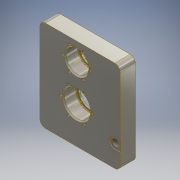
# Autodesk Inventor part: корпус_02
Saved by Autodesk Inventor 2016 (Build 200138000, 138)
## iProperties
Created: 2021-04-26
Part Number: корпус_02
Material: Типовые
Document SubType Name: Modeling
Designer: Лол
Density: 1 g/cm^3
Appearance: Титан — полированный
Author: Лол
Autodesk Inventor part; units mm, degrees
ref_plane "YZ Plane" through (0, 0, 0) normal (1, 0, 0) x (0, 1, 0)
ref_plane "XY Plane" through (0, 0, 0) normal (0, 0, 1) x (1, 0, 0)
ref_plane "РабПлоскость1" through (0, -12.5, 0) normal (0, 1, 0) x (-1, 0, 0)
sketch "Эскиз2" plane through (0, -12.5, 0) normal (0, 1, 0) x (-1, 0, 0)
  line L0 (100, 120) -> (-120, 120)
  line L1 (-120, 120) -> (-120, -130)
  line L2 (-120, -130) -> (100, -130)
  line L3 (100, -130) -> (100, 120)
  line L4 (144, 0) -> (-164, 0) projected
  line L5 (-164, 0) -> (144, 0) projected
  line L6 (0, -180) -> (0, 170) projected
  circle A0 centre (0, 70) radius 27
  circle A1 centre (0, -30) radius 31.5
  point P0 (0, 0)
  dimension "d10" = 120
  dimension "d11" = 130
  dimension "d12" = 120
  dimension "d13" = 100
  dimension "d14" = 70
  dimension "d15" = 30
  dimension "d16" = 63
  dimension "d17" = 54
  constraints: 8 end point, 2 centre point, 2 parallel, 2 point on line, 1 horizontal, 1 perpendicular
  measures "d10" distance between parallel lines of L4 L0
  measures "d11" distance between parallel lines of L2 L4
  measures "d12" distance between parallel lines of L6 L1
  measures "d13" distance between parallel lines of L3 L6
  measures "d14" distance from line of L4 A0.centre
  measures "d15" distance from line of A1.centre L4
  measures "d16" diameter of A1
  measures "d17" diameter of A0
extrude "Выдавливание2" add sketch "Эскиз2" against normal blind 42 contours L3 L4 A1 L6 A0 L0 | L6 A0 A1 L4 L1 L0 | L3 L2 L6 A1 L4 | L4 A1 L6 L2 L1
fillet "Сопряжение1" radius 15 4 edges at (120, -33.5, 120) (120, -33.5, -130) (-100, -33.5, 120) (-100, -33.5, -130)
sketch "Эскиз3" plane through (0, -12.5, 0) normal (0, 1, 0) x (1, 0, 0)
  line L0 (-85, -120) -> (105, -120) projected
  arc A0 (-100, -105) -> (-85, -120) centre (-85, -105) ccw construction
  line L1 (-100, 115) -> (-100, -105) projected
  arc A1 (-85, 130) -> (-100, 115) centre (-85, 115) ccw construction
  arc A2 (120, 115) -> (105, 130) centre (105, 115) ccw projected
  line L2 (120, -105) -> (120, 115) projected
  arc A3 (105, -120) -> (120, -105) centre (105, -105) ccw projected
  arc A4 (-85, 130) -> (-100, 115) centre (-85, 115) ccw projected
  line L3 (-100, 115) -> (-100, -105) projected
  arc A5 (-100, -105) -> (-85, -120) centre (-85, -105) ccw projected
  line L4 (-85, -120) -> (105, -120) projected
  arc A6 (105, -120) -> (120, -105) centre (105, -105) ccw projected
  line L5 (120, -105) -> (120, 115) projected
  arc A7 (120, 115) -> (105, 130) centre (105, 115) ccw projected
  line L6 (105, 130) -> (-85, 130) construction
  circle A8 centre (0, 30) radius 31.5 projected
  circle A9 centre (0, -70) radius 27 projected
  circle A10 centre (0, 30) radius 31.5 projected
  arc A11 (-94, -105) -> (-85, -114) centre (-85, -105) ccw
  arc A12 (105, -114) -> (114, -105) centre (105, -105) ccw
  line L7 (114, -105) -> (114, 115)
  arc A13 (114, 115) -> (105, 124) centre (105, 115) ccw
  line L8 (105, 124) -> (-85, 124)
  arc A14 (-85, 124) -> (-94, 115) centre (-85, 115) ccw
  line L9 (-94, 115) -> (-94, -105)
  arc A15 (27.534, -11.7358) -> (-27.534, -11.7358) centre (0, 30) ccw
  arc A16 (35.3716, -97.8182) -> (26.8965, -33.9226) centre (0, -70) ccw
  arc A17 (-26.8965, -33.9226) -> (-35.3716, -97.8182) centre (0, -70) ccw
  arc A18 (-26.8965, -33.9226) -> (-27.534, -11.7358) centre (-35.0001, -23.0529) ccw
  arc A19 (27.534, -11.7358) -> (26.8965, -33.9226) centre (35.0001, -23.0529) ccw
  line L10 (168.3492, 0) -> (-148.3492, 0) projected
  line L11 (0, 184.3492) -> (0, -174.3492) projected
  line L12 (-85, -114) -> (-43.2319, -114)
  line L13 (43.2319, -114) -> (105, -114)
  arc A20 (-43.2319, -114) -> (-35.3716, -97.8182) centre (-43.2319, -104) ccw
  arc A21 (35.3716, -97.8182) -> (43.2319, -114) centre (43.2319, -104) ccw
  point P0 (0, 0)
  dimension "d21" = 6
  dimension "d22" = 100
  dimension "d24" = 45
  dimension "d25" = 45
  dimension "d27" = 13.558
  dimension "d28" = 6
  dimension "d32" = 10
  dimension "d33" = 10
  dimension "d34" = 238
  dimension "d35" = 114
  dimension "d38" = 114
  constraints: 22 point on circle, 11 centre point, 10 end point, 9 tangent, 2 coincident, 1 equal radius, 3 other
  measures "d21" distance between parallel lines of L1 L9
  measures "d22" diameter of A15
  measures "d24" radius of A17
  measures "d25" radius of A16
  measures "d27" radius of A18
  measures "d28" distance between parallel lines of L0 L13
  measures "d32" radius of A20
  measures "d33" radius of A21
  measures "d34" distance between parallel lines of L12 L8
  measures "d35" distance between parallel lines of L11 L7
  measures "d38" distance between parallel lines of L10 L12
extrude "Выдавливание5" cut sketch "Эскиз3" against normal blind 34 contours L10 A15 A18 A17 A20 L12 A11 L9 | L9 A14 L8 L11 A15 L10 | L10 A15 L11 L8 A13 L7 | L7 A12 L13 A21 A16 A19 A15 L10
sketch "Эскиз4" plane through (0, -54.5, 0) normal (0, -1, 0) x (1, 0, 0)
  circle A0 centre (0, -30) radius 31.5 projected
  circle A1 centre (0, 70) radius 27 projected
  arc A2 (-100, -115) -> (-85, -130) centre (-85, -115) ccw projected
  line L0 (-85, -130) -> (105, -130) projected
  arc A3 (105, -130) -> (120, -115) centre (105, -115) ccw projected
  line L1 (120, -115) -> (120, 105) projected
  arc A4 (120, 105) -> (105, 120) centre (105, 105) ccw projected
  line L2 (105, 120) -> (-85, 120) projected
  arc A5 (-85, 120) -> (-100, 105) centre (-85, 105) ccw projected
  line L3 (-100, 105) -> (-100, -115) projected
  circle A6 centre (0, 70) radius 31
  circle A7 centre (0, -30) radius 36
  circle A8 centre (0, -30) radius 31.5
  circle A9 centre (0, 70) radius 27
  point P0 (0, 0)
  dimension "d41" = 62
  dimension "d42" = 72
  constraints: 4 centre point, 4 coincident, 2 concentric
  measures "d41" diameter of A6
  measures "d42" diameter of A7
extrude "Выдавливание7" cut sketch "Эскиз4" against normal blind 37 contours A6 | A7
sketch "Эскиз5" plane through (0, -12.5, 0) normal (0, 1, 0) x (1, 0, 0)
  arc A0 (105, -120) -> (120, -105) centre (105, -105) ccw projected
  arc A1 (-100, -105) -> (-85, -120) centre (-85, -105) ccw projected
  arc A2 (-85, 130) -> (-100, 115) centre (-85, 115) ccw projected
  arc A3 (120, 115) -> (105, 130) centre (105, 115) ccw projected
  arc A4 (-70, 115) -> (-94, 103) centre (-85, 115) ccw
  circle A5 centre (-85, -105) radius 15
  arc A6 (114, 103) -> (90, 115) centre (105, 115) ccw
  circle A7 centre (105, -105) radius 15
  line L0 (105, -114) -> (43.2319, -114) projected
  line L1 (114, 115) -> (114, -105) projected
  arc A8 (-94, -105) -> (-85, -114) centre (-85, -105) ccw projected
  line L2 (-43.2319, -114) -> (-85, -114) projected
  arc A9 (-43.2319, -114) -> (-35.3716, -97.8182) centre (-43.2319, -104) ccw projected
  arc A10 (-26.8965, -33.9226) -> (-35.3716, -97.8182) centre (0, -70) ccw projected
  arc A11 (-26.8965, -33.9226) -> (-27.534, -11.7358) centre (-35.0001, -23.0529) ccw projected
  arc A12 (27.534, -11.7358) -> (-27.534, -11.7358) centre (0, 30) ccw projected
  arc A13 (27.534, -11.7358) -> (26.8965, -33.9226) centre (35.0001, -23.0529) ccw projected
  arc A14 (35.3716, -97.8182) -> (26.8965, -33.9226) centre (0, -70) ccw projected
  arc A15 (35.3716, -97.8182) -> (43.2319, -114) centre (43.2319, -104) ccw projected
  line L3 (105, -114) -> (43.2319, -114) projected
  arc A16 (105, -114) -> (114, -105) centre (105, -105) ccw projected
  line L4 (114, 115) -> (114, -105) projected
  arc A17 (114, 115) -> (105, 124) centre (105, 115) ccw projected
  line L5 (-85, 124) -> (105, 124) projected
  arc A18 (-85, 124) -> (-94, 115) centre (-85, 115) ccw projected
  line L6 (-94, -105) -> (-94, 115) projected
  line L7 (-85, 124) -> (105, 124) projected
  line L8 (-94, -105) -> (-94, 115) projected
  line L9 (-43.2319, -114) -> (-85, -114) projected
  line L10 (-70, 115) -> (-70, 65)
  arc A19 (-94, 53) -> (-70, 65) centre (-85, 65) ccw
  line L11 (-100, 115) -> (-100, -105) projected
  line L12 (90, 115) -> (90, 65)
  arc A20 (90, 65) -> (114, 53) centre (105, 65) ccw
  line L13 (105, 65) -> (105, 115) construction
  line L14 (120, -105) -> (120, 115) projected
  point P0 (0, 0)
  dimension "d117" = 50
  dimension "d118" = 50
  constraints: 8 point on circle, 6 centre point, 6 end point, 6 equal radius, 4 coincident, 4 point on line, 3 vertical, 2 tangent, 1 parallel
  measures "d117" distance of L10.end L10.start
  measures "d118" distance of A2.centre A19.centre
extrude "Выдавливание8" add sketch "Эскиз5" against normal blind 37 contours A7 L0 A16 L1 A0 | A7 L1 A16 L0 | A6 L1 A17 L5 A3 | A20 L12 A6 L5 A17 L1 | L5 A18 L6 A4 A2 | A4 L10 A19 L6 A18 L5 | A5 L6 A8 L2 A1 | A5 L2 A8 L6
fillet "Сопряжение2" radius 15 2 edges at (-73, -29.5, 114) (93, -29.5, -124)
fillet "Сопряжение3" radius 5 6 edges at (114, -29.5, 93) (93, -29.5, 114) (-94, -29.5, 93) (-73, -29.5, -124) (-94, -29.5, -53) (114, -29.5, -53)
sketch "Эскиз6" plane through (0, -12.5, 0) normal (0, 1, 0) x (1, 0, 0)
  line L0 (85.4041, -114) -> (43.2319, -114) projected
  arc A0 (35.3716, -97.8182) -> (43.2319, -114) centre (43.2319, -104) ccw projected
  arc A1 (35.3716, -97.8182) -> (26.8965, -33.9226) centre (0, -70) ccw projected
  arc A2 (27.534, -11.7358) -> (26.8965, -33.9226) centre (35.0001, -23.0529) ccw projected
  arc A3 (27.534, -11.7358) -> (-27.534, -11.7358) centre (0, 30) ccw projected
  arc A4 (-26.8965, -33.9226) -> (-27.534, -11.7358) centre (-35.0001, -23.0529) ccw projected
  arc A5 (-26.8965, -33.9226) -> (-35.3716, -97.8182) centre (0, -70) ccw projected
  arc A6 (-43.2319, -114) -> (-35.3716, -97.8182) centre (-43.2319, -104) ccw projected
  line L1 (-43.2319, -114) -> (-55.6061, -114) projected
  arc A7 (-70.3031, -102) -> (-55.6061, -114) centre (-55.6061, -99) ccw projected
  arc A8 (-70.3031, -102) -> (-88, -90.3031) centre (-85, -105) ccw projected
  arc A9 (-94, -85.4041) -> (-88, -90.3031) centre (-89, -85.4041) ccw projected
  line L2 (-94, -85.4041) -> (-94, 45.4041) projected
  arc A10 (-70, 115) -> (-70.3031, 118) centre (-85, 115) ccw projected
  arc A11 (-65.4041, 124) -> (-70.3031, 118) centre (-65.4041, 119) ccw projected
  line L3 (-65.4041, 124) -> (75, 124) projected
  arc A12 (90, 109) -> (75, 124) centre (75, 109) ccw projected
  line L4 (114, 45.4041) -> (114, -85.4041) projected
  arc A13 (108, -90.3031) -> (114, -85.4041) centre (109, -85.4041) ccw projected
  arc A14 (108, -90.3031) -> (90.3031, -108) centre (105, -105) ccw projected
  arc A15 (85.4041, -114) -> (90.3031, -108) centre (85.4041, -109) ccw projected
  circle A16 centre (0, -70) radius 27 projected
  circle A17 centre (0, 30) radius 31.5 projected
  arc A18 (105, -120) -> (120, -105) centre (105, -105) ccw projected
  line L5 (120, -105) -> (120, 115) projected
  arc A19 (120, 115) -> (105, 130) centre (105, 115) ccw projected
  line L6 (105, 130) -> (-85, 130) projected
  arc A20 (-85, 130) -> (-100, 115) centre (-85, 115) ccw projected
  line L7 (-100, 115) -> (-100, -105) projected
  arc A21 (-100, -105) -> (-85, -120) centre (-85, -105) ccw projected
  line L8 (-85, -120) -> (105, -120) projected
  arc A22 (108, -90.3031) -> (90.3031, -108) centre (105, -105) ccw projected
  arc A23 (-70.3031, -102) -> (-88, -90.3031) centre (-85, -105) ccw projected
  arc A24 (-70.3031, 118) -> (-70.3031, 118) centre (-85, 115) ccw projected
  circle A25 centre (95, 120) radius 1.5
  circle A26 centre (-75, -110) radius 1.5
  arc A27 (-88, 50.3031) -> (-70, 65) centre (-85, 65) ccw projected
  line L9 (-70, 65) -> (-70, 115) projected
  line L10 (90, 109) -> (90, 65) projected
  arc A28 (90, 65) -> (108, 50.3031) centre (105, 65) ccw projected
  arc A29 (-88, 50.3031) -> (-94, 45.4041) centre (-89, 45.4041) ccw projected
  arc A30 (114, 45.4041) -> (108, 50.3031) centre (109, 45.4041) ccw projected
  point P0 (0, 0)
  point P1 (-88, 100.3031)
  dimension "d51" = 5
  dimension "d52" = 10
  dimension "d55" = 3
  dimension "d56" = 3
  constraints: 2 centre point, 1 other
  measures "d51" vertical distance of A8.centre A26.centre
  measures "d52" horizontal distance of A26.centre A8.centre
  measures "d55" diameter of A25
  measures "d56" diameter of A26
hole "Отверстие1" at (95, -12.5, -120) at (-75, -12.5, 110) direction (0, -1, 0) diameter 6 depth 10 tip angle 118 countersink diameter 7.2 countersink angle 90
sketch "Эскиз7" plane through (0, -12.5, 0) normal (0, 1, 0) x (1, 0, 0)
  arc A0 (-100, -105) -> (-85, -120) centre (-85, -105) ccw projected
  circle A1 centre (95, 120) radius 3.6 projected
  circle A2 centre (-75, -110) radius 3.6 projected
  line L0 (85.4041, -114) -> (43.2319, -114) projected
  arc A3 (35.3716, -97.8182) -> (43.2319, -114) centre (43.2319, -104) ccw projected
  arc A4 (35.3716, -97.8182) -> (26.8965, -33.9226) centre (0, -70) ccw projected
  arc A5 (27.534, -11.7358) -> (26.8965, -33.9226) centre (35.0001, -23.0529) ccw projected
  arc A6 (27.534, -11.7358) -> (-27.534, -11.7358) centre (0, 30) ccw projected
  arc A7 (-26.8965, -33.9226) -> (-27.534, -11.7358) centre (-35.0001, -23.0529) ccw projected
  arc A8 (-26.8965, -33.9226) -> (-35.3716, -97.8182) centre (0, -70) ccw projected
  arc A9 (-43.2319, -114) -> (-35.3716, -97.8182) centre (-43.2319, -104) ccw projected
  line L1 (-43.2319, -114) -> (-55.6061, -114) projected
  arc A10 (-70.3031, -102) -> (-55.6061, -114) centre (-55.6061, -99) ccw projected
  arc A11 (-70.3031, -102) -> (-88, -90.3031) centre (-85, -105) ccw projected
  arc A12 (-94, -85.4041) -> (-88, -90.3031) centre (-89, -85.4041) ccw projected
  line L2 (-94, -85.4041) -> (-94, 45.4041) projected
  arc A13 (-70, 115) -> (-70.3031, 118) centre (-85, 115) ccw projected
  arc A14 (-65.4041, 124) -> (-70.3031, 118) centre (-65.4041, 119) ccw projected
  line L3 (-65.4041, 124) -> (75, 124) projected
  arc A15 (90, 109) -> (75, 124) centre (75, 109) ccw projected
  line L4 (114, 45.4041) -> (114, -85.4041) projected
  arc A16 (108, -90.3031) -> (114, -85.4041) centre (109, -85.4041) ccw projected
  arc A17 (108, -90.3031) -> (90.3031, -108) centre (105, -105) ccw projected
  arc A18 (85.4041, -114) -> (90.3031, -108) centre (85.4041, -109) ccw projected
  circle A19 centre (0, -70) radius 27 projected
  circle A20 centre (0, 30) radius 31.5 projected
  arc A21 (105, -120) -> (120, -105) centre (105, -105) ccw projected
  line L5 (120, -105) -> (120, 115) projected
  arc A22 (120, 115) -> (105, 130) centre (105, 115) ccw projected
  line L6 (105, 130) -> (-85, 130) projected
  arc A23 (-85, 130) -> (-100, 115) centre (-85, 115) ccw projected
  line L7 (-100, 115) -> (-100, -105) projected
  arc A24 (-100, -105) -> (-85, -120) centre (-85, -105) ccw projected
  line L8 (-85, -120) -> (105, -120) projected
  arc A25 (120, 115) -> (105, 130) centre (105, 115) ccw projected
  arc A26 (105, -120) -> (120, -105) centre (105, -105) ccw projected
  arc A27 (-88, 50.3031) -> (-70, 65) centre (-85, 65) ccw projected
  line L9 (-70, 65) -> (-70, 115) projected
  line L10 (90, 109) -> (90, 65) projected
  arc A28 (90, 65) -> (108, 50.3031) centre (105, 65) ccw projected
  arc A29 (-88, 50.3031) -> (-94, 45.4041) centre (-89, 45.4041) ccw projected
  arc A30 (114, 45.4041) -> (108, 50.3031) centre (109, 45.4041) ccw projected
  point P0 (0, 0)
hole "Отверстие2" at (-85, -12.5, -115) at (-85, -12.5, 105) at (105, -12.5, 105) at (105, -12.5, -115) direction (0, -1, 0) diameter 8.647 depth 23 tip angle 118 countersink diameter 12 countersink angle 90 thread size "M10x1.25" class "6H" standard "ISO Metric profile"
chamfer "Фаска1" distance 3.3 angle 45 1 edges at (-36, -54.5, -30)
chamfer "Фаска2" distance 3.3 angle 45 1 edges at (-31, -54.5, 70)
sketch "Эскиз8" plane through (0, -54.5, 0) normal (0, -1, 0) x (1, 0, 0)
  circle A0 centre (0, -30) radius 31.5 projected
  circle A1 centre (0, -30) radius 36 projected
  circle A2 centre (0, -30) radius 42.5 construction
  line L0 (-144, 0) -> (164, 0) projected
  line L1 (0, 170) -> (0, -180) projected
  line L2 (0, -30) -> (-42.5, -30) construction
  circle A3 centre (-42.5, -30) radius 1
  circle A4 centre (-21.25, -66.8061) radius 1
  circle A5 centre (21.25, -66.8061) radius 1
  circle A6 centre (42.5, -30) radius 1
  circle A7 centre (21.25, 6.8061) radius 1
  circle A8 centre (-21.25, 6.8061) radius 1
  point P0 (0, 0)
  dimension "d77" = 85
  dimension "d78" = 2
  dimension "d81" = 360
  constraints: 7 centre point, 2 end point, 2 point on circle, 1 coincident, 13 other
  measures "d77" diameter of A2
  measures "d78" diameter of A3
hole "Отверстие3" at (-42.5, -54.5, -30) at (-21.25, -54.5, -66.8061) at (21.25, -54.5, -66.8061) at (42.5, -54.5, -30) at (21.25, -54.5, 6.8061) at (-21.25, -54.5, 6.8061) direction (0, 1, 0) diameter 4.917 depth 15 tip angle 118 countersink diameter 7.2 countersink angle 90 thread size "M6x1" class "6H" standard "ISO Metric profile"
sketch "Эскиз9" plane through (0, 0, 0) normal (1, 0, 0) x (0, 1, 0)
  point P0 (0, 0)
sketch "Эскиз10" plane through (0, 0, 0) normal (1, 0, 0) x (0, 1, 0)
  line L0 (-17.5, 39) -> (-17.5, 101) projected
  line L1 (-51.2, 39) -> (-17.5, 39) projected
  line L2 (-51.2, 6) -> (-17.5, 6) projected
  line L3 (-17.5, -66) -> (-17.5, 6) projected
  line L4 (-20.45, 39) -> (-20.2, 38.75)
  line L5 (-20.2, 38.75) -> (-17.2, 38.75)
  line L6 (-17.2, 38.75) -> (-17.2, 41.75)
  line L7 (-17.2, 41.75) -> (-17.5, 42.05)
  line L8 (-20.45, 6) -> (-20.2, 6.25)
  line L9 (-20.2, 6.25) -> (-17.2, 6.25)
  line L10 (-17.2, 6.25) -> (-17.2, 3.25)
  line L11 (-17.2, 3.25) -> (-17.5, 2.95)
  line L12 (-65.4, -30) -> (10.9, -30) projected
  line L13 (-65.4, 70) -> (10.9, 70) projected
  point P0 (0, 0)
  dimension "d90" = 45
  dimension "d91" = 45
  dimension "d92" = 3
  dimension "d93" = 0.25
  dimension "d94" = 0.3
  dimension "d95" = 45
  dimension "d96" = 45
  dimension "d97" = 3
  dimension "d98" = 0.25
  dimension "d99" = 0.3
  constraints: 16 end point, 4 perpendicular, 4 point on line, 2 horizontal
  measures "d90" angle of L0 L7
  measures "d91" angle of L1 L4
  measures "d92" distance of L4.end L5.end
  measures "d93" distance between parallel lines of L1 L5
  measures "d94" distance between parallel lines of L0 L6
  measures "d95" angle of L2 L8
  measures "d96" angle of L3 L11
  measures "d97" distance of L8.end L9.end
  measures "d98" distance between parallel lines of L2 L9
  measures "d99" distance between parallel lines of L3 L10
revolve "Вращение1" cut sketch "Эскиз10" angle 360 about axis through (0, -54.5, -30) along (0, 1, 0) contours L8 L9 L10 L11 L3 L2
revolve "Вращение2" cut sketch "Эскиз10" angle 360 about axis through (0, -54.5, 70) along (0, 1, 0) contours L0 L7 L6 L5 L4 L1
fillet "Сопряжение4" radius 1 2 edges at (0, -17.2, 101.25) (0, -17.2, -66.25)
fillet "Сопряжение5" radius 0.5 4 edges at (0, -20.2, 101.25) (0, -17.2, 98.25) (0, -20.2, -66.25) (0, -17.2, -63.25)
sketch "Эскиз11" plane through (0, -54.5, 0) normal (0, -1, 0) x (1, 0, 0)
  circle A0 centre (0, 70) radius 31 projected
  circle A1 centre (0, 70) radius 31 projected
  circle A2 centre (0, 70) radius 37.5 construction
  line L0 (0, 70) -> (-37.5, 70) construction
  line L1 (0, 170) -> (0, -180) projected
  line L2 (-144, 0) -> (164, 0) projected
  circle A3 centre (-37.5, 70) radius 3
  point P0 (0, 0)
  dimension "d104" = 75
  dimension "d106" = 6
  constraints: 2 coincident, 2 end point, 1 centre point, 1 horizontal, 1 horizontal alignment, 2 other
  measures "d106" diameter of A3
hole "Отверстие4" at (-37.5, -54.5, 70) direction (0, 1, 0) diameter 4.917 depth 15.1 tip angle 118 countersink diameter 7.2 countersink angle 90 thread size "M6x1" class "6H" standard "ISO Metric profile"
pattern_circular "Круговой массив1" count 6 over 360 about axis through (0, -54.5, 70) along (0, 1, 0) of "Отверстие4"
sketch "Эскиз12" plane through (-100, -12.5, -115) normal (-1, 0, 0) x (0, 0, 1)
  line L0 (0, -42) -> (0, 0) projected
  line L1 (0, 0) -> (220, 0) projected
  line L2 (220, -42) -> (0, -42) projected
  line L3 (-6, 0) -> (6, 0) projected
  line L4 (64.6969, -34) -> (64.6969, 0) projected
  circle A0 centre (34.6969, -21) radius 13
  line L5 (34.6969, -21) -> (34.6969, 0) construction
  line L6 (34.6969, -21) -> (34.6969, -42) construction
  point P0 (115, 12.5)
  dimension "d121" = 26
  dimension "d124" = 30
  constraints: 4 end point, 2 perpendicular, 2 point on line, 1 centre point, 1 collinear
  measures "d121" diameter of A0
  measures "d124" distance from line of L4 L5.start
hole "Отверстие5" at (-100, -33.5, -80.3031) direction (1, 0, 0) diameter 18.376 end up to face face through (-70, -35.1667, -98.3333) facing (1, 0, 0) counterbore diameter 30 counterbore depth 2 thread size "M20x1.5" class "6H" standard "ISO Metric profile"
fillet "Сопряжение6" radius 5 27 edges at (-92.1623, -46.5, -49.2771) (-75.5132, -46.5, -53.381) (-70, -46.5, -90) (-70.076, -46.5, -116.5076) (-69.2771, -46.5, -122.1623) (4.798, -46.5, -124) (85.6066, -46.5, -119.6066) (90, -46.5, -87) (95.5132, -46.5, -53.381) (112.1623, -46.5, -49.2771) (114, -46.5, 20) (112.1623, -46.5, 89.2771) (94.3934, -46.5, 94.3934) (89.2771, -46.5, 112.1623) (64.318, -46.5, 114) (34.237, -46.5, 108.3693) (44.6093, -46.5, 64.083) (21.4477, -46.5, 22.6635) (0, -46.5, -80) (-21.4477, -46.5, 22.6635) (-44.6093, -46.5, 64.083) (-34.237, -46.5, 108.3693) (-49.419, -46.5, 114) (-65.093, -46.5, 110.619) (-76.729, -46.5, 92.4864) (-92.1623, -46.5, 89.2771) (-94, -46.5, 20)
sketch "Эскиз13" plane through (0, -54.5, 0) normal (0, -1, 0) x (1, 0, 0)
  line L0 (120, -115) -> (120, 105) projected
  arc A0 (105, -130) -> (120, -115) centre (105, -115) ccw projected
  line L1 (-85, -130) -> (105, -130) projected
  line L2 (90, -109) -> (90, -65) projected
  arc A1 (108, -50.3031) -> (90, -65) centre (105, -65) ccw projected
  arc A2 (108, -50.3031) -> (114, -45.4041) centre (109, -45.4041) ccw projected
  arc A3 (75, -124) -> (90, -109) centre (75, -109) ccw projected
  line L3 (114, -45.4041) -> (114, 85.4041) projected
  circle A4 centre (105, -70) radius 10
  line L4 (105, -115) -> (105, -65) construction
  point P0 (0, 0)
  dimension "d133" = 20
  dimension "d134" = 45
  constraints: 2 end point, 1 centre point, 1 point on line, 1 vertical
  measures "d133" diameter of A4
  measures "d134" distance of A4.centre L4.start
hole "Отверстие6" at (105, -54.5, -70) direction (0, 1, 0) diameter 18.376 end through all counterbore diameter 30 counterbore depth 2 thread size "M20x1.5" class "6H" standard "ISO Metric profile"
ref_plane "РабПлоскость2" through (-65.4041, -12.5, -46.25) normal (0, 0, 1) x (1, 0, 0)
sketch "Эскиз15" plane through (0, -54.5, 0) normal (0, -1, 0) x (1, 0, 0)
  circle A0 centre (105, -70) radius 15 projected
  line L0 (120, 105) -> (120, -115) projected
  line L1 (105, -85) -> (120, -85)
  line L2 (105, -55) -> (120, -55)
  point P0 (0, 0)
  point P1 (120, -70)
  constraints: 4 end point, 2 perpendicular, 2 point on circle, 2 point on line, 2 tangent
extrude "Выдавливание10" cut sketch "Эскиз15" against normal blind 2 contours L0 L1 A0 | A0 L2 L0
sketch "Эскиз14" plane through (-65.4041, -12.5, -46.25) normal (0, 0, 1) x (1, 0, 0)
  line L0 (179.5921, -42) -> (161.2161, -42) projected
  line L1 (161.2161, -1.7) -> (179.5921, -1.7) projected
  line L2 (161.2161, 0) -> (161.2161, -40) projected
  line L3 (174.7276, -23) -> (174.7276, -1.6765) projected
  line L4 (179.5921, 0) -> (179.5921, -40) projected
  line L5 (170.4041, -42) -> (170.4041, 0) projected
  circle A0 centre (174.5921, -17) radius 5
  point P0 (65.4041, 12.5)
  dimension "d145" = 10
  dimension "d146" = 5
  dimension "d147" = 25
  constraints: 1 centre point, 2 other
  measures "d145" diameter of A0
  measures "d146" distance from line of L4 A0.centre
